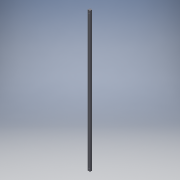
# Autodesk Inventor part: HSR20-xxxx-01
Saved by Autodesk Inventor 2016 SP1 (Build 200210100, 210)
## iProperties
Created: 2014-08-19
Part Number: HSR20-xxxx-01
Cost Center: 0 kg
Material: Steel
Document SubType Name: Modeling
Designer: Gaspoz
Authority: 0 mm^3
Mass: 223.276 g
Surface Area: 91.6942 cm^2
Volume: 28.4428 cm^3
Density: 7.85 g/cm^3
Catalog Web Link: gaspoz.free.fr/TLWXPN
Description: THK Caged Ball LM Guide
Appearance: Steel
Data_di_Salvataggio: 2007-01-24
Ora_di_salvataggio: 13.40
Massa_totale: 0 kg
Volume_totale: 0 mm^3
Author: Gaspoz
Autodesk Inventor part; units mm, degrees
ref_plane "YZ Plane" through (0, 0, 0) normal (1, 0, 0) x (0, 1, 0)
ref_plane "XZ Plane" through (0, 0, 0) normal (0, 1, 0) x (-1, 0, 0)
ref_plane "XY Plane" through (0, 0, 0) normal (0, 0, 1) x (1, 0, 0)
sketch "Sketch4" plane through (0, 0, 0) normal (0, 0, 1) x (1, 0, 0)
  line L0 (10, 4.0001) -> (10, 1)
  line L1 (6.55, 7.45) -> (10, 4.0001)
  line L2 (6.55, 10.3792) -> (6.55, 7.45)
  line L3 (7.7659, 11.5951) -> (6.55, 10.3792)
  arc A0 (9.4852, 13.3144) -> (7.7659, 11.5951) centre (9.8015, 11.2788) ccw
  line L4 (10, 13.8292) -> (9.4852, 13.3144)
  line L5 (10, 15.16) -> (10, 13.8292)
  line L6 (9.4727, 15.6874) -> (10, 15.16)
  arc A1 (7.7679, 17.3921) -> (9.4727, 15.6874) centre (9.8015, 17.7209) ccw
  line L7 (7.16, 18) -> (7.7679, 17.3921)
  line L8 (-7.16, 18) -> (7.16, 18)
  line L9 (-7.7679, 17.3921) -> (-7.16, 18)
  arc A2 (-9.4727, 15.6874) -> (-7.7679, 17.3921) centre (-9.8015, 17.7209) ccw
  line L10 (-10, 15.16) -> (-9.4727, 15.6874)
  line L11 (-10, 13.8292) -> (-10, 15.16)
  line L12 (-9.4852, 13.3144) -> (-10, 13.8292)
  arc A3 (-7.7659, 11.5951) -> (-9.4852, 13.3144) centre (-9.8015, 11.2788) ccw
  line L13 (-6.55, 10.3792) -> (-7.7659, 11.5951)
  line L14 (-6.55, 7.45) -> (-6.55, 10.3792)
  line L15 (-10, 4.0001) -> (-6.55, 7.45)
  line L16 (-10, 1) -> (-10, 4.0001)
  line L17 (-9, 0) -> (-10, 1)
  line L18 (-3, 0) -> (-9, 0)
  line L19 (-2.5, 0.5) -> (-3, 0)
  line L20 (2.5, 0.5) -> (-2.5, 0.5)
  line L21 (3, 0) -> (2.5, 0.5)
  line L22 (9, 0) -> (3, 0)
  line L23 (10, 1) -> (9, 0)
  point P0 (0, 0)
  point P1 (0, 0)
  constraints: 48 end point, 8 point on circle, 4 centre point
extrude "Extrusion4" add sketch "Sketch4" along normal mid plane 1060
sketch "Sketch5" plane through (-7.16, 18, 530) normal (0, 1, 0) x (1, 0, 0)
  line L0 (0, 0) -> (14.3201, 0) projected
  line L1 (0, 1060) -> (0, 0) projected
  line L2 (7.16, 0) -> (7.16, 20)
  point P0 (7.16, 530)
  dimension "d8" = 20
  constraints: 2 end point, 1 midpoint, 1 parallel
  measures "d8" distance of L2.start L2.end
hole "Hole1" at (0, 18, 510) direction (0, -1, 0) diameter 6 end through all counterbore diameter 9.5 counterbore depth 8.5
pattern_linear "Rectangular Pattern1" count 2 spacing 1020 along (0, 0, -1) of "Hole1"
equation "\"d6\" = L"
equation "\"d8\" = testa"
equation "\"d18\" = passo"
equation "\"passo\" = 1020"
equation "\"testa\" = 20"
equation "\"L\" = 1060"
body "Solid1"
